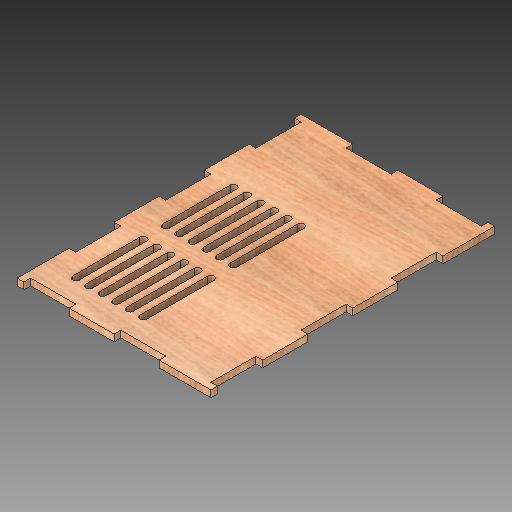
# Autodesk Inventor part: ControlBoxTop
Saved by Autodesk Inventor 2018.2 (Build 222227000, 227)
## iProperties
Created: 2018-03-30
Part Number: ControlBoxTop
Material: Wood (Birch)
Document SubType Name: Modeling
Designer: Muchen He
Density: 0.55 g/cm^3
Appearance: Birch - Natural Polished
Mass: 14.9674 g
Surface Area: 220.936 cm^2
Volume: 27.2135 cm^3
Author: Muchen He
Autodesk Inventor part; units mm, degrees
ref_plane "YZ Plane" through (0, 0, 0) normal (1, 0, 0) x (0, 1, 0)
ref_plane "XZ Plane" through (0, 0, 0) normal (0, 1, 0) x (-1, 0, 0)
ref_plane "XY Plane" through (0, 0, 0) normal (0, 0, 1) x (1, 0, 0)
sketch "Sketch1" plane through (0, 0, 0) normal (0, 1, 0) x (-1, 0, 0)
  line L0 (0, 0) -> (-80, 0)
  line L1 (-80, 0) -> (-80, -120)
  line L2 (-80, -120) -> (0, -120)
  line L3 (0, -120) -> (0, 0)
  line L4 (0, -120) -> (0, -123)
  line L5 (0, -123) -> (-20, -123)
  line L6 (-20, -123) -> (-20, -120)
  line L7 (-40, -123) -> (-60, -123)
  line L8 (-60, -123) -> (-60, -120)
  line L9 (-40, -120) -> (-40, -123)
  line L10 (-80, 0) -> (-80, 3)
  line L11 (-80, 3) -> (-60, 3)
  line L12 (-60, 3) -> (-60, 0)
  line L13 (-40, 3) -> (-20, 3)
  line L14 (-40, 0) -> (-40, 3)
  line L15 (-20, 3) -> (-20, 0)
  line L16 (0, 0) -> (3, 0)
  line L17 (3, 0) -> (3, -20)
  line L18 (3, -20) -> (0, -20)
  line L19 (3, -60) -> (0, -60)
  line L20 (3, -40) -> (3, -60)
  line L21 (0, -40) -> (3, -40)
  line L22 (3, -100) -> (0, -100)
  line L23 (3, -80) -> (3, -100)
  line L24 (0, -80) -> (3, -80)
  line L25 (-80, -120) -> (-83, -120)
  line L26 (-83, -120) -> (-83, -100)
  line L27 (-83, -100) -> (-80, -100)
  line L28 (-83, -60) -> (-80, -60)
  line L29 (-83, -80) -> (-83, -60)
  line L30 (-80, -80) -> (-83, -80)
  line L31 (-83, -20) -> (-80, -20)
  line L32 (-83, -40) -> (-83, -20)
  line L33 (-80, -40) -> (-83, -40)
  line L34 (0, -20) -> (0, -40)
  line L35 (0, -60) -> (0, -80)
  line L36 (0, -100) -> (0, -123)
  line L37 (-20, -120) -> (-40, -120)
  line L38 (-60, -120) -> (-83, -120)
  line L39 (-80, -100) -> (-80, -80)
  line L40 (-80, -60) -> (-80, -40)
  line L41 (-80, -20) -> (-80, 3)
  line L42 (-60, 0) -> (-40, 0)
  line L43 (-20, 0) -> (3, 0)
  line L44 (-80, 3) -> (-83, 3)
  line L45 (-83, 3) -> (-83, 0)
  line L46 (-83, 0) -> (-80, 0)
  line L47 (3, 0) -> (3, 3)
  line L48 (3, 3) -> (0, 3)
  line L49 (0, 3) -> (0, 0)
  line L50 (0, -120) -> (3, -120)
  line L51 (3, -120) -> (3, -123)
  line L52 (3, -123) -> (0, -123)
  line L53 (-80, -120) -> (-80, -123)
  line L54 (-80, -123) -> (-83, -123)
  line L55 (-83, -123) -> (-83, -120)
  dimension "d0" = 120
  dimension "d1" = 80
  dimension "d2" = 3
  dimension "d3" = 20
  dimension "d13" = 40
  dimension "d18" = 3
  dimension "d19" = 20
  dimension "d22" = 40
  dimension "d27" = 3
  dimension "d28" = 20
  dimension "d31" = 40
  dimension "d36" = 3
  dimension "d37" = 20
  dimension "d40" = 40
  dimension "d47" = 3
  dimension "d48" = 3
  dimension "d49" = 3
  constraints: 112 end point, 18 perpendicular, 9 collinear, 7 horizontal, 6 vertical, 4 point on line, 2 parallel, 1 vertical alignment, 42 other
  measures "d0" distance of L2.end L0.start
  measures "d1" distance of L1.end L2.end
  measures "d2" distance of L2.end L4.end
  measures "d3" distance of L4.end L5.end
  measures "d13" distance of L4.end L7.start
  measures "d18" distance of L0.end L10.end
  measures "d19" distance of L10.end L11.end
  measures "d22" distance of L10.end L13.start
  measures "d27" distance of L0.start L16.end
  measures "d28" distance of L16.end L17.end
  measures "d31" distance of L17.end L19.start
  measures "d36" distance of L1.end L25.end
  measures "d37" distance of L25.end L26.end
  measures "d40" distance of L26.end L28.start
  measures "d47" distance of L16.end L47.end
  measures "d48" distance of L2.end L50.end
  measures "d49" distance of L54.end L25.end
extrude "Extrusion3" add sketch "Sketch1" along normal blind 3
sketch "Sketch2" plane through (0, 3, 0) normal (0, 1, 0) x (1, 0, 0)
  line L0 (10, 10) -> (10, 40) construction
  line L1 (11.5, 10) -> (11.5, 40)
  line L2 (8.5, 40) -> (8.5, 10)
  arc A0 (8.5, 10) -> (11.5, 10) centre (10, 10) ccw
  arc A1 (11.5, 40) -> (8.5, 40) centre (10, 40) ccw
  line L3 (0, 40) -> (0, 20) projected
  line L4 (0, 0) -> (20, 0) projected
  point P0 (10, 25)
  dimension "d50" = 30
  dimension "d51" = 3
  dimension "d52" = 10
  dimension "d53" = 10
  constraints: 8 end point, 4 point on circle, 4 tangent, 2 centre point, 1 midpoint, 1 parallel, 1 vertical
  measures "d50" distance of L0.start L0.end
  measures "d51" diameter of A1
  measures "d52" distance from line of L3 L0.start
  measures "d53" distance from line of L4 L0.start
extrude "Extrusion4" cut sketch "Sketch2" against normal up to next
pattern_linear "Rectangular Pattern2" count 2 spacing 40 along (0, 0, -1) of "Extrusion4"
pattern_linear "Rectangular Pattern3" count 6 spacing 6 along (1, 0, 0) of "Extrusion4", "Rectangular Pattern2"
body "Solid2"
